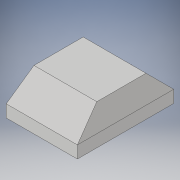
# Autodesk Inventor part: Sensor
Saved by Autodesk Inventor 2019 (Build 230136000, 136)
## iProperties
Created: 2020-02-01
Part Number: Sensor
Material: Generic
Document SubType Name: Modeling
Designer: alb16148
Density: 1 g/cm^3
Appearance: Default
Author: alb16148
Autodesk Inventor part; units mm, degrees
ref_plane "YZ Plane" through (0, 0, 0) normal (1, 0, 0) x (0, 1, 0)
ref_plane "XZ Plane" through (0, 0, 0) normal (0, 1, 0) x (-1, 0, 0)
ref_plane "XY Plane" through (0, 0, 0) normal (0, 0, 1) x (1, 0, 0)
sketch "Sketch1" plane through (0, 0, 0) normal (0, 1, 0) x (-1, 0, 0)
  line L0 (1.51, 2.045) -> (-1.51, 2.045)
  line L1 (-1.51, 2.045) -> (-1.51, -2.045)
  line L2 (-1.51, -2.045) -> (1.51, -2.045)
  line L3 (1.51, -2.045) -> (1.51, 2.045)
  point P0 (0, 0)
  dimension "d0" = 1.51
  dimension "d1" = 1.51
  dimension "d2" = 2.045
  dimension "d3" = 2.045
  constraints: 8 end point, 2 parallel, 1 horizontal, 1 perpendicular
  measures "d0" distance from line of L3 point (0, 0)
  measures "d1" distance from line of point (0, 0) L1
  measures "d2" distance from line of point (0, 0) L0
  measures "d3" distance from line of point (0, 0) L2
extrude "Extrusion1" add sketch "Sketch1" along normal blind 1.52
chamfer "Chamfer1" distance 1 angle 45 2 edges at (0, 1.52, 2.045) (0, 1.52, -2.045) measured on face at (0.5033, 1.52, 0.6817)
chamfer "Chamfer2" distance 1 angle 10 1 edges at (-1.51, 1.52, 0) measured on face at (-1.51, 0.5067, -0.3483)
chamfer "Chamfer3" distance 1 angle 10 1 edges at (1.51, 1.52, 0) measured on face at (1.51, 0.5067, 0.3483)
equation "\"d1\" = d0"
equation "\"d3\" = d2"
body "Solid1"
